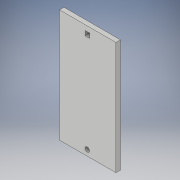
# Autodesk Inventor part: Lclamp1
Saved by Autodesk Inventor 2019 (Build 230136000, 136)
## iProperties
Created: 2020-02-26
Part Number: Lclamp1
Material: Generic
Document SubType Name: Modeling
Designer: Hp
Density: 1 g/cm^3
Appearance: Default
Author: Hp
Autodesk Inventor part; units mm, degrees
ref_plane "YZ Plane" through (0, 0, 0) normal (1, 0, 0) x (0, 1, 0)
ref_plane "XZ Plane" through (0, 0, 0) normal (0, 1, 0) x (-1, 0, 0)
ref_plane "XY Plane" through (0, 0, 0) normal (0, 0, 1) x (1, 0, 0)
sketch "Sketch1" plane through (0, 0, 0) normal (0, 0, 1) x (1, 0, 0)
  line L0 (-12.2998, 27.0657) -> (12.7002, 27.0657)
  line L1 (12.7002, 27.0657) -> (12.7002, -22.9343)
  line L2 (12.7002, -22.9343) -> (-12.2998, -22.9343)
  line L3 (-12.2998, -22.9343) -> (-12.2998, 27.0657)
  circle A0 centre (0, -20.3589) radius 1
  line L4 (-0.9186, 24.8477) -> (1.0814, 24.8477)
  line L5 (1.0814, 24.8477) -> (1.0814, 22.8477)
  line L6 (1.0814, 22.8477) -> (-0.9186, 22.8477)
  line L7 (-0.9186, 22.8477) -> (-0.9186, 24.8477)
  point P0 (0, 0)
  dimension "d0" = 25
  dimension "d1" = 50
  dimension "d2" = 2
  dimension "d3" = 2
  dimension "d4" = 2
  constraints: 16 end point, 4 parallel, 2 horizontal, 2 perpendicular, 1 centre point
  measures "d0" distance of L1.end L2.end
  measures "d1" distance of L0.end L1.end
  measures "d2" diameter of A0
  measures "d3" distance of L5.end L6.end
  measures "d4" distance of L4.end L5.end
extrude "Extrusion1" add sketch "Sketch1" along normal blind 2
body "Solid1"
